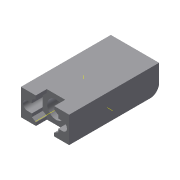
# Autodesk Inventor part: empty
Saved by Autodesk Inventor 2014 (Build 180170000, 170)
## iProperties
Created: 2015-04-13
Part Number: empty
Material: Generic
Document SubType Name: Modeling
Designer: Martin
Density: 1 g/cm^3
Appearance: Default
Mass: 0.578402 g
Surface Area: 7.54528 cm^2
Volume: 0.578402 cm^3
Author: Martin
Autodesk Inventor part; units mm, degrees
ref_plane "plane_support" through (-5.5, -7.5, -3) normal (0, -1, 0) x (1, 0, 0)
ref_plane "plane_support_frontb" through (-2.75, 0, 0) normal (1, 0, 0) x (0, 0, -1)
ref_plane "plane_support_frontt" through (2.75, 0, 0) normal (-1, 0, 0) x (0, 0, 1)
sketch "Sketch14" plane through (0, 0, 0) normal (1, 0, 0) x (0, 1, 0)
  line L0 (-12.85, 0) -> (15.85, 0) projected
  line L1 (0, -4.2) -> (0, 4.2) projected
  line L2 (8.75, -3) -> (-8.75, -3)
  line L3 (-8.75, -3) -> (-8.75, 3)
  line L4 (-8.75, 3) -> (8.75, 3)
  line L5 (8.75, 3) -> (8.75, -3) construction
  line L6 (8.75, -3) -> (-8.75, 3) construction
  line L7 (-8.75, -3) -> (8.75, 3) construction
  line L8 (5.25, 3) -> (5.25, -3) construction
  line L9 (-6.25, 3) -> (-6.25, -3) construction
  arc A0 (8.75, -3) -> (8.75, 3) centre (8.75, 0) ccw
  circle A1 centre (8.75, 0) radius 1.25 construction
  circle A2 centre (8.75, 0) radius 3 construction
  line L10 (5.75, 3) -> (5.75, -3) construction
  line L11 (11.75, 3) -> (11.75, -3)
  line L12 (11.75, -3) -> (8.75, -3)
  line L13 (8.75, 3) -> (11.75, 3)
  point P0 (0, 0)
  point P1 (0, 0)
  dimension "d72" = 6
  dimension "d74" = 2.5
  dimension "d75" = 2.5
  dimension "d76" = 0.5
  dimension "d105" = 18
  constraints: 24 end point, 8 tangent, 6 point on line, 5 perpendicular, 4 parallel, 3 centre point, 3 midpoint, 2 coincident, 2 point on circle, 1 concentric, 1 horizontal
  measures "d72" distance between parallel lines of L2 L4
  measures "d74" distance between parallel lines of L3 L9
  measures "d75" diameter of A1
  measures "d76" distance between parallel lines of L8 L10
  measures "d105" distance between parallel lines of L11 L9
extrude "ext_main" add sketch "Sketch14" along normal mid plane 11
sketch "sk_channel_nut" plane through (-5.5, -8.75, -3) normal (0, -1, 0) x (1, 0, 0)
  line L0 (-2.2, 3) -> (13.2, 3) projected
  line L1 (5.5, -1.8497) -> (5.5, 7.8497) projected
  circle A0 centre (5.5, 3) radius 2
  line L2 (5.5, 6.4641) -> (2.5, 4.7321)
  line L3 (2.5, 4.7321) -> (2.5, 1.2679)
  line L4 (2.5, 1.2679) -> (5.5, -0.4641)
  line L5 (5.5, -0.4641) -> (8.5, 1.2679)
  line L6 (8.5, 1.2679) -> (8.5, 4.7321)
  line L7 (8.5, 4.7321) -> (5.5, 6.4641)
  circle A1 centre (1.5, 3) radius 1
  circle A2 centre (9.5, 3) radius 1
  line L8 (1.5, 4) -> (2.5, 4)
  line L9 (1.5, 2) -> (2.5, 2)
  line L10 (9.5, 4) -> (8.5, 4)
  line L11 (9.5, 2) -> (8.5, 2)
  line L12 (0, 0) -> (11, 0) projected
  line L13 (0, 6) -> (11, 6) projected
  line L14 (0, 0) -> (0, 6) projected
  line L15 (3.4, 6) -> (3.4, 5.2517)
  line L16 (3.4456, 0.722) -> (3.4456, 0)
  line L17 (7.5544, 0.722) -> (7.5544, 0)
  line L18 (7.6, 6) -> (7.6, 5.2517)
  point P0 (2.5, 3)
  dimension "d85" = 4
  dimension "d86" = 120
  dimension "d87" = 6
  dimension "d88" = 2
  dimension "d95" = 4.2
  constraints: 28 end point, 17 point on line, 7 parallel, 5 equal length, 5 point on circle, 5 tangent, 3 centre point, 3 perpendicular, 1 coincident, 1 equal radius, 1 midpoint, 2 other
  measures "d85" diameter of A0
  measures "d86" angle of L7 L2
  measures "d87" distance between parallel lines of L3 L6
  measures "d88" diameter of A1
  measures "d95" distance between parallel lines of L18 L15
extrude "ext_cut_channel" cut sketch "sk_channel_nut" against normal through all contours A0 L1 L0 | L0 L1 A0 | L1 A0 L0 | L0 A0 L1
extrude "ext_cut_bottomscrews" cut sketch "sk_channel_nut" against normal blind 8 contours A1 L0 | L0 A1 | A1 L8 L3 | L3 L9 A1 | A2 L0 | A2 L11 L6 | L6 L10 A2 | L0 A2
extrude "ext_cut_bottom_nut" cut sketch "sk_channel_nut" against normal blind 2.5 contours L3 L2 L13 L1 A0 L0 | L0 A0 L1 L12 L4 L3 | L16 L4 L12 | L13 L2 L15 | A0 L1 L0 | L0 L1 A0 | L12 L1 L4 | L2 L1 L13 | L1 A0 L0 | L0 A0 L1 | L1 L13 L7 L6 L0 A0 | A0 L0 L6 L5 L12 L1 | L1 L12 L5 | L7 L13 L1 | L5 L17 L12 | L13 L18 L7
fillet "Fillet1" radius 2 1 edges at (0, 11.75, -3)
sketch "Sketch19" plane through (-5.5, -7.5, -3) normal (0, -1, 0) x (1, 0, 0)
  line L0 (3.4, 6) -> (7.6, 6) projected
  line L1 (3.4, 5.2517) -> (3.4, 6) projected
  line L2 (2.5, 4.7321) -> (3.4, 5.2517) projected
  line L3 (2.5, 4) -> (2.5, 4.7321) projected
  line L4 (2.5, 2) -> (2.5, 4) projected
  line L5 (2.5, 1.2679) -> (2.5, 2) projected
  line L6 (3.4456, 0.722) -> (2.5, 1.2679) projected
  line L7 (3.4456, 0) -> (3.4456, 0.722) projected
  line L8 (7.5544, 0) -> (3.4456, 0) projected
  line L9 (7.5544, 0.722) -> (7.5544, 0) projected
  line L10 (8.5, 1.2679) -> (7.5544, 0.722) projected
  line L11 (8.5, 2) -> (8.5, 1.2679) projected
  line L12 (8.5, 4) -> (8.5, 2) projected
  line L13 (8.5, 4.7321) -> (8.5, 4) projected
  line L14 (7.6, 5.2517) -> (8.5, 4.7321) projected
  line L15 (7.6, 6) -> (7.6, 5.2517) projected
  circle A0 centre (5.5, 3) radius 2 projected
  line L16 (3.65, 5.75) -> (7.35, 5.75) construction
  line L17 (7.35, 5.75) -> (7.35, 5.1073)
  line L18 (7.35, 5.1073) -> (8.25, 4.5877)
  line L19 (8.25, 4.5877) -> (8.25, 4)
  line L20 (8.25, 4) -> (8.25, 2)
  line L21 (8.25, 2) -> (8.25, 1.4123)
  line L22 (8.25, 1.4123) -> (7.3044, 0.8664)
  line L23 (7.3044, 0.8664) -> (7.3044, 0.25)
  line L24 (7.3044, 0.25) -> (3.6956, 0.25) construction
  line L25 (3.6956, 0.25) -> (3.6956, 0.8664)
  line L26 (3.6956, 0.8664) -> (2.75, 1.4123)
  line L27 (2.75, 1.4123) -> (2.75, 2)
  line L28 (2.75, 2) -> (2.75, 4)
  line L29 (2.75, 4) -> (2.75, 4.5877)
  line L30 (2.75, 4.5877) -> (3.65, 5.1073)
  line L31 (3.65, 5.1073) -> (3.65, 5.75)
  line L32 (3.65, 5.75) -> (7.35, 5.75)
  line L33 (7.35, 5.75) -> (7.35, 6)
  line L34 (7.35, 6) -> (3.65, 6)
  line L35 (3.65, 6) -> (3.65, 5.75)
  line L36 (3.6956, 0.25) -> (7.3044, 0.25)
  line L37 (7.3044, 0.25) -> (7.3044, 0)
  line L38 (7.3044, 0) -> (3.6956, 0)
  line L39 (3.6956, 0) -> (3.6956, 0.25)
  point P0 (5.5, 3)
  dimension "d97" = 0.25
  constraints: 48 end point, 6 equal length, 2 collinear, 2 perpendicular, 15 other
  measures "d97" horizontal distance of L16.start L0.start
sketch "Sketch20" plane through (-2.75, 0, 0) normal (1, 0, 0) x (0, 0, -1)
  circle A0 centre (0, 9) radius 1.25 projected
  arc A1 (3, 9) -> (-3, 9) centre (0, 9) ccw projected
  line L0 (-3, 6) -> (-3, 9) projected
  line L1 (3, 6) -> (-3, 6) projected
  line L2 (3, 9) -> (3, 6) projected
  line L3 (-3, 7) -> (3, 7)
  point P0 (0, 0)
  dimension "d102" = 1
  constraints: 2 end point, 2 point on line, 1 perpendicular
  measures "d102" distance between parallel lines of L1 L3
equation "\"d74\" = nut_m3_thickness_max"
equation "\"d75\" = screw_m2_bore_loose"
equation "\"d87\" = nut_m3_width_acrossflats"
equation "\"d88\" = screw_m2_bore_selfthreading"
equation "\"d95\" = 0.7 * nut_m3_width_acrossflats"
equation "\"d89\" = linact_rod_effective_length + nut_m3_thickness_max"
equation "\"d93\" = nut_m3_thickness_max"
equation "\"d97\" = print_support_z_clearance"
equation "\"d102\" = print_support_xy_clearance"
equation "\"d96\" = print_support_xy_clearance"
equation "\"d100\" = print_support_z_clearance"
equation "\"d101\" = print_support_z_clearance"
equation "\"nut_m3_thickness_max\" = 2.5"
equation "\"screw_m2_bore_loose\" = 2.5"
equation "\"nut_m3_width_acrossflats\" = 6"
equation "\"screw_m2_bore_selfthreading\" = 2"
equation "\"linact_rod_effective_length\" = 12"
equation "\"print_support_z_clearance\" = 0.25"
equation "\"print_support_xy_clearance\" = 1"
body "Solid3"
